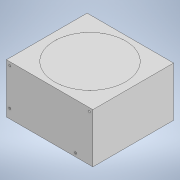
# Autodesk Inventor part: PSU
Saved by Autodesk Inventor 2021 (Build 250183000, 183)
## iProperties
Created: 2022-01-08
Part Number: PSU
Material: Generic
Document SubType Name: Modeling
Designer: ipodk
Density: 1 g/cm^3
Appearance: Default
Author: ipodk
Autodesk Inventor part; units mm, degrees
ref_plane "YZ Plane" through (0, 0, 0) normal (1, 0, 0) x (0, 1, 0)
ref_plane "XZ Plane" through (0, 0, 0) normal (0, 1, 0) x (-1, 0, 0)
ref_plane "XY Plane" through (0, 0, 0) normal (0, 0, 1) x (1, 0, 0)
sketch "Sketch1" plane through (0, 0, 0) normal (0, 1, 0) x (-1, 0, 0)
  line L0 (0, 0) -> (150, 0)
  line L1 (150, 0) -> (150, -140)
  line L2 (150, -140) -> (0, -140)
  line L3 (0, -140) -> (0, 0)
  dimension "d0" = 140
  dimension "d2" = 150
  constraints: 8 end point, 2 parallel, 1 horizontal, 1 perpendicular
  measures "d0" distance of L0.end L1.end
  measures "d2" distance between parallel lines of L3 L1
extrude "Extrusion1" add sketch "Sketch1" along normal blind 86
sketch "Sketch2" plane through (-150, 0, 0) normal (0, 0, 1) x (1, 0, 0)
  line L0 (150, 0) -> (0, 0) projected
  line L1 (0, 0) -> (6, 0)
  line L2 (6, 0) -> (6, 16)
  line L3 (6, 16) -> (6, 80)
  line L4 (6, 80) -> (144, 80)
  line L5 (0, 0) -> (0, 86) projected
  line L6 (6, 80) -> (144, 80) construction
  circle A0 centre (6, 16) radius 1.75
  line L7 (120, 0) -> (120, 6)
  circle A1 centre (120, 6) radius 1.75
  circle A2 centre (6, 80) radius 1.75
  circle A3 centre (144, 80) radius 1.75
  dimension "d5" = 6
  dimension "d6" = 16
  dimension "d7" = 64
  dimension "d8" = 138
  dimension "d9" = 360
  dimension "d10" = 6
  dimension "d11" = 114
  dimension "d12" = 74
  dimension "d13" = 3.5
  dimension "d14" = 3.5
  dimension "d15" = 3.5
  dimension "d16" = 3.5
  constraints: 12 end point, 4 centre point, 4 coincident, 3 vertical, 2 point on line, 1 collinear, 1 horizontal, 1 perpendicular
  measures "d5" distance of L0.end L1.end
  measures "d6" distance of L1.end L2.end
  measures "d7" distance of L2.end L3.end
  measures "d8" distance of L3.end L4.end
  measures "d10" distance of L7.start L7.end
  measures "d11" distance between parallel lines of L7 L2
  measures "d12" distance from line of L7.end L4
  measures "d13" diameter of A2
  measures "d14" diameter of A0
  measures "d15" diameter of A1
  measures "d16" diameter of A3
extrude "Extrusion2" cut sketch "Sketch2" against normal blind 4.7625
sketch "Sketch3" plane through (0, 86, 0) normal (0, 1, 0) x (1, 0, 0)
  line L0 (-150, 140) -> (-150, 0) projected
  line L1 (-150, 140) -> (-75, 140)
  line L2 (-75, 140) -> (-75, 70)
  line L3 (-75, 70) -> (-150, 70)
  line L4 (-150, 70) -> (-150, 140)
  line L5 (0, 0) -> (0, 140) projected
  line L6 (-150, 140) -> (0, 140)
  line L7 (0, 140) -> (0, 0)
  line L8 (0, 0) -> (-150, 0)
  line L9 (-150, 0) -> (-150, 140)
  circle A0 centre (-75, 70) radius 61.5476
  dimension "d19" = 70
  dimension "d20" = 140
  dimension "d21" = 150
  dimension "d22" = 75
  constraints: 16 end point, 4 parallel, 2 horizontal, 2 perpendicular, 1 centre point, 1 coincident
  measures "d19" distance of L1.end L2.end
  measures "d20" distance of L5.start L5.end
  measures "d21" distance of L5.start L8.end
  measures "d22" distance of L2.end L3.end
extrude "Extrusion3" cut sketch "Sketch3" against normal blind 0.01 contours A0 L2 L3 | L3 L2 A0
equation "\"d14\" = d13"
equation "\"d15\" = d13"
equation "\"d16\" = d13"
equation "\"d19\" = 0.5 * d20"
equation "\"d22\" = 0.5 * d21"
body "Solid1"
